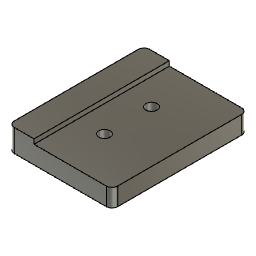
Espaçador PDU (Autodesk Fusion 360 design; units mm, degrees)
Autodesk Fusion 360 part; units mm, degrees
sketch "Sketch1" plane through (0, 0, 0) normal (0, 0, 1) x (1, 0, 0)
  line L0 (0, 0) -> (55, 0)
  line L1 (55, 0) -> (55, 72)
  line L2 (55, 72) -> (0, 72)
  line L3 (0, 72) -> (0, 0)
  circle A0 centre (27.5, 23.5) radius 3
  line L4 (0, 36) -> (55, 36) construction
  circle A1 centre (27.5, 48.5) radius 3
  dimension "d1" = 55
  dimension "d2" = 72
  dimension "d8" = 6
  dimension "d9" = 25
  constraint horizontal L0
  constraint vertical L1
  constraint horizontal L2
  constraint vertical L3
  constraint coincident L0.start L3.end
  constraint midpoint L3 L4.start
  constraint midpoint L1 L4.end
  constraint symmetric A0 L4 A1
  measures "d1" distance of L0.start L0.end
  measures "d2" distance of L0.start L2.end
  measures "d8" diameter of A0
  measures "d9" distance of A0.centre A1.centre
extrude "Extrude1" add sketch "Sketch1" along normal blind 12
sketch "Sketch2" plane through (0, 0, 12) normal (0, 0, 1) x (-1, 0, 0)
  line L0 (0, -72) -> (0, 0)
  line L1 (0, 0) -> (-55, 0)
  line L2 (-55, 0) -> (-55, -72)
  line L3 (-55, -72) -> (0, -72)
  line L4 (-13.5, 0) -> (-13.5, -72)
  circle A0 centre (-27.5, -23.5) radius 3
  circle A1 centre (-27.5, -48.5) radius 3
  dimension "d5" = 13.5
  constraint coincident L1 L4.start
  constraint coincident L3 L4.end
  constraint perpendicular L3 L4
  measures "d5" distance of L0 L4
extrude "Extrude2" cut sketch "Sketch2" against normal blind 2.5 contours L1 L2 L3 L4 | A0 | A1
fillet "Fillet1" radius 3 4 edges at (0, 0, 6) (55, 0, 4.75) (55, 72, 4.75) (0, 72, 6)
named bodies: "Espaçador PDU"
